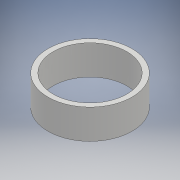
# Autodesk Inventor part: base-ring
Saved by Autodesk Inventor 2018 (Build 220112000, 112)
## iProperties
Created: 2019-09-09
Part Number: base-ring
Material: Generic
Document SubType Name: Modeling
Designer: dsikar
Density: 1 g/cm^3
Appearance: Default
Author: dsikar
Autodesk Inventor part; units mm, degrees
ref_plane "YZ Plane" through (0, 0, 0) normal (1, 0, 0) x (0, 1, 0)
ref_plane "XZ Plane" through (0, 0, 0) normal (0, 1, 0) x (-1, 0, 0)
ref_plane "XY Plane" through (0, 0, 0) normal (0, 0, 1) x (1, 0, 0)
sketch "Sketch1" plane through (0, 0, 0) normal (0, 1, 0) x (-1, 0, 0)
  line L0 (8.7, 0) -> (9.9, 0)
  line L1 (9.9, 0) -> (9.9, 7)
  line L2 (9.9, 7) -> (8.7, 7)
  line L3 (8.7, 7) -> (8.7, 0)
  line L4 (0, -1.4) -> (0, 8.4) projected
  point P0 (0, 0)
  dimension "d0" = 1.2
  dimension "d1" = 7
  dimension "d2" = 8.7
  constraints: 8 end point, 2 parallel, 1 horizontal, 1 perpendicular
  measures "d0" distance of L2.end L1.end
  measures "d1" distance of L1.end L0.end
  measures "d2" distance from line of L3 point (0, 0)
revolve "Revolution1" add sketch "Sketch1" angle 360 about axis through (0, 0, -10) along (0, 0, 1)
body "Solid1"
